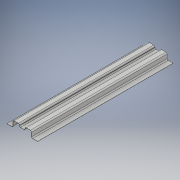
# Autodesk Inventor part: AAD0001106802
Saved by Autodesk Inventor 2017 (Build 210142000, 142)
## iProperties
Created: 2019-04-10
Part Number: AAD0001106802
Material: Generic
Document SubType Name: Modeling
Designer: Phs
Density: 1 g/cm^3
Appearance: Default
Author: Phs
Autodesk Inventor part; units mm, degrees
ref_plane "YZ Plane" through (0, 0, 0) normal (1, 0, 0) x (0, 1, 0)
ref_plane "XZ Plane" through (0, 0, 0) normal (0, 1, 0) x (-1, 0, 0)
ref_plane "XY Plane" through (0, 0, 0) normal (0, 0, 1) x (1, 0, 0)
sketch "Sketch1" plane through (0, 0, 0) normal (0, 0, 1) x (1, 0, 0)
  line L0 (-41.8, 0) -> (-61.75, 0)
  line L1 (-15.75, 24.3) -> (-33, 24.3)
  line L2 (0, 14.3) -> (-6.95, 14.3)
  line L3 (-11.75, 20.3) -> (-11.75, 19.1)
  line L4 (-37, 20.3) -> (-37, 4.8)
  arc A0 (-11.75, 19.1) -> (-6.95, 14.3) centre (-6.95, 19.1) ccw
  arc A1 (-11.75, 20.3) -> (-15.75, 24.3) centre (-15.75, 20.3) ccw
  arc A2 (-33, 24.3) -> (-37, 20.3) centre (-33, 20.3) ccw
  arc A3 (-41.8, 0) -> (-37, 4.8) centre (-41.8, 4.8) ccw
  line L5 (-61.75, 0.8) -> (-41.8, 0.8)
  arc A4 (-41.8, 0.8) -> (-37.8, 4.8) centre (-41.8, 4.8) ccw
  line L6 (-37.8, 4.8) -> (-37.8, 20.3)
  arc A5 (-33, 25.1) -> (-37.8, 20.3) centre (-33, 20.3) ccw
  line L7 (-33, 25.1) -> (-15.75, 25.1)
  arc A6 (-10.95, 20.3) -> (-15.75, 25.1) centre (-15.75, 20.3) ccw
  line L8 (-10.95, 20.3) -> (-10.95, 19.1)
  arc A7 (-10.95, 19.1) -> (-6.95, 15.1) centre (-6.95, 19.1) ccw
  line L9 (-6.95, 15.1) -> (0, 15.1)
  line L10 (-61.75, 0) -> (-61.75, 0.8)
  line L11 (0, 0) -> (0, 9.3563)
  line L12 (0, 14.3) -> (0, 15.1)
  dimension "d0" = 14.3
  dimension "d2" = 24.3
  dimension "d4" = 25.25
  dimension "d5" = 4.8
  dimension "d6" = 4
  dimension "d8" = 0.8
  dimension "d11" = 6.95
  dimension "d12" = 19.95
  constraints: 26 end point, 16 point on circle, 8 centre point, 8 tangent, 3 horizontal, 2 equal radius, 2 parallel, 2 vertical, 1 perpendicular, 1 point on line, 8 other
  measures "d0" distance of L11.start L2.start
  measures "d2" distance between parallel lines of L1 L0
  measures "d4" distance between parallel lines of L3 L4
  measures "d5" radius of A0
  measures "d6" radius of A1
  measures "d8" distance between parallel lines of L4 L6
  measures "d11" distance of L2.start L2.end
  measures "d12" distance of L0.start L0.end
extrude "Extrusion1" add sketch "Sketch1" along normal mid plane 545
mirror "Mirror1" about plane through (0, 0, 0) normal (1, 0, 0) of "Extrusion1"
body "Solid1"
